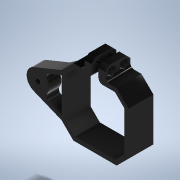
# Autodesk Inventor part: Montura motor para cadena
Saved by Autodesk Inventor 2022 (Build 260153000, 153)
## iProperties
Created: 2022-02-14
Part Number: Montura motor para cadena
Material: PET Plastic
Document SubType Name: Modeling
Designer: juanp
Density: 1.541 g/cm^3
Appearance: Polycarbonate - Clear
Author: juanp
Autodesk Inventor part; units mm, degrees
ref_plane "YZ Plane" through (0, 0, 0) normal (1, 0, 0) x (0, 1, 0)
ref_plane "XZ Plane" through (0, 0, 0) normal (0, 1, 0) x (-1, 0, 0)
ref_plane "XY Plane" through (0, 0, 0) normal (0, 0, 1) x (1, 0, 0)
sketch "Sketch1" plane through (0, 0, 0) normal (0, 0, 1) x (1, 0, 0)
  line L0 (21.15, -21.15) -> (14.4175, -21.15) construction
  line L1 (-21.15, -21.15) -> (-21.15, -14.4175) construction
  line L2 (-21.15, 21.15) -> (-14.4175, 21.15) construction
  line L3 (21.15, 21.15) -> (21.15, 14.4175) construction
  line L4 (21.15, -21.15) -> (-21.15, 21.15) construction
  line L5 (-21.15, -21.15) -> (21.15, 21.15) construction
  line L6 (-21.15, 14.4175) -> (-14.4175, 21.15) construction
  line L7 (14.4175, 21.15) -> (21.15, 14.4175) construction
  line L8 (21.15, -14.4175) -> (14.4175, -21.15) construction
  line L9 (-14.4175, -21.15) -> (-21.15, -14.4175) construction
  line L10 (-21.15, 14.4175) -> (-21.15, 21.15) construction
  line L11 (-14.4175, 21.15) -> (14.4175, 21.15) construction
  line L12 (14.4175, 21.15) -> (21.15, 21.15) construction
  line L13 (21.15, 14.4175) -> (21.15, -14.4175) construction
  line L14 (21.15, -14.4175) -> (21.15, -21.15) construction
  line L15 (14.4175, -21.15) -> (-14.4175, -21.15) construction
  line L16 (-14.4175, -21.15) -> (-21.15, -21.15) construction
  line L17 (-21.15, -14.4175) -> (-21.15, 14.4175) construction
  line L18 (-21.25, 14.4589) -> (-14.4589, 21.25)
  line L19 (-14.4589, 21.25) -> (14.4589, 21.25)
  line L20 (14.4589, 21.25) -> (21.25, 14.4589)
  line L21 (21.25, 14.4589) -> (21.25, -14.4589)
  line L22 (21.25, -14.4589) -> (14.4589, -21.25)
  line L23 (14.4589, -21.25) -> (-14.4589, -21.25)
  line L24 (-14.4589, -21.25) -> (-21.25, -14.4589)
  line L25 (-21.25, -14.4589) -> (-21.25, 14.4589)
  line L26 (-24.25, 15.7015) -> (-15.7015, 24.25)
  line L27 (-15.7015, 24.25) -> (15.7015, 24.25)
  line L28 (15.7015, 24.25) -> (24.25, 15.7015)
  line L29 (24.25, 15.7015) -> (24.25, -15.7015)
  line L30 (24.25, -15.7015) -> (15.7015, -24.25)
  line L31 (15.7015, -24.25) -> (-15.7015, -24.25)
  line L32 (-15.7015, -24.25) -> (-24.25, -15.7015)
  line L33 (-24.25, -15.7015) -> (-24.25, 15.7015)
  line L34 (-7.5, 21.25) -> (-2.5, 21.25)
  line L35 (-2.5, 21.25) -> (-2.5, 33.25)
  line L36 (-2.5, 33.25) -> (-7.5, 33.25)
  line L37 (-7.5, 33.25) -> (-7.5, 21.25)
  line L38 (2.5, 21.25) -> (7.5, 21.25)
  line L39 (7.5, 21.25) -> (7.5, 33.25)
  line L40 (7.5, 33.25) -> (2.5, 33.25)
  line L41 (2.5, 33.25) -> (2.5, 21.25)
  line L42 (-2.5, 27.25) -> (2.5, 27.25) construction
  line L43 (0, 27.25) -> (0, 21.15) construction
  point P0 (0, 0)
  point P1 (-17.7837, -17.7837)
  point P2 (-17.7837, 17.7837)
  point P3 (17.7837, 17.7837)
  point P4 (17.7837, -17.7837)
  point P5 (-7.5, 24.25)
  point P6 (7.5, 24.25)
  dimension "d0" = 42.3
  dimension "d1" = 42.3
  dimension "d2" = 50.3
  dimension "d3" = 0.1
  dimension "d4" = 3
  dimension "d5" = 5
  dimension "d6" = 5
  dimension "d7" = 9
  constraints: 88 end point, 26 parallel, 13 perpendicular, 10 midpoint, 9 point on line, 5 horizontal, 4 equal length, 1 collinear, 1 vertical, 14 other
  measures "d0" distance of L2.start L3.start
  measures "d1" distance of L1.start L2.start
  measures "d2" distance between parallel lines of L6 L8
  measures "d3" distance between parallel lines of L17 L25
  measures "d4" distance between parallel lines of L25 L33
  measures "d5" distance of L39.end L40.end
  measures "d6" distance between parallel lines of L41 L35
  measures "d7" distance between parallel lines of L40 L27
extrude "Extrusion1" add sketch "Sketch1" along normal blind 18 contours L25 L24 L23 L22 L21 L20 L19 L39 L27 L28 L29 L30 L31 L32 L33 L26 L37 L18 | L37 L27 L35 L19 | L37 L36 L35 L27 | L41 L27 L39 L19 | L41 L40 L39 L27
sketch "Sketch2" plane through (7.5, 24.25, 0) normal (1, 0, 0) x (0, 0, -1)
  line L0 (0, 0) -> (0, 9) projected
  line L1 (0, 9) -> (-18, 9) projected
  line L2 (-18, 0) -> (-18, 9) projected
  line L3 (0, 0) -> (-18, 0) projected
  line L4 (-18, 4.5) -> (-13.5, 4.5) construction
  line L5 (-4.5, 4.5) -> (0, 4.5) construction
  line L6 (0, 9) -> (0, -3) projected
  circle A0 centre (-13.5, 4.5) radius 1.65
  circle A1 centre (-4.5, 4.5) radius 1.65
  line L7 (-13.5, 4.5) -> (-9, 4.5) construction
  line L8 (-9, 4.5) -> (-4.5, 4.5) construction
  line L9 (-13.5, 1.2553) -> (-16.31, 2.8776)
  line L10 (-16.31, 2.8776) -> (-16.31, 6.1224)
  line L11 (-16.31, 6.1224) -> (-13.5, 7.7447)
  line L12 (-13.5, 7.7447) -> (-10.69, 6.1224)
  line L13 (-10.69, 6.1224) -> (-10.69, 2.8776)
  line L14 (-10.69, 2.8776) -> (-13.5, 1.2553)
  line L15 (-1.69, 2.8776) -> (-4.5, 1.2553)
  line L16 (-4.5, 1.2553) -> (-7.31, 2.8776)
  line L17 (-7.31, 2.8776) -> (-7.31, 6.1224)
  line L18 (-7.31, 6.1224) -> (-4.5, 7.7447)
  line L19 (-4.5, 7.7447) -> (-1.69, 6.1224)
  line L20 (-1.69, 6.1224) -> (-1.69, 2.8776)
  circle A2 centre (-13.5, 4.5) radius 4.5
  circle A3 centre (-4.5, 4.5) radius 4.5
  point P0 (0, -24.25)
  point P1 (-4.5, 0)
  point P2 (-13.5, 0)
  point P3 (-4.5, 9)
  point P4 (-13.5, 9)
  dimension "d10" = 3.3
  dimension "d11" = 5.62
  constraints: 32 end point, 5 coincident, 4 equal length, 3 point on line, 2 centre point, 2 horizontal, 2 vertical, 1 collinear, 1 equal radius, 1 midpoint, 1 perpendicular, 32 other
  measures "d10" diameter of A0
  measures "d11" distance between parallel lines of L10 L13
extrude "Extrusion2" cut sketch "Sketch2" against normal blind 15 contours A0 | A1
extrude "Extrusion4" cut sketch "Sketch2" against normal blind 2.35 contours L9 L10 L11 L12 L13 L14 | L15 L16 L17 L18 L19 L20
fillet "Fillet1" radius 3 4 edges at (-7.5, 24.25, 9) (2.5, 21.25, 9) (-2.5, 21.25, 9) (7.5, 24.25, 9)
chamfer "Chamfer1" distance 3 angle 45 4 edges at (-5, 33.25, 0) (5, 33.25, 0) (-5, 33.25, 18) (5, 33.25, 18)
ref_plane "Work Plane1" through (0, 0, 9) normal (0, 0, -1) x (-1, 0, 0)
sketch "Sketch3" plane through (0, 0, 9) normal (0, 0, 1) x (1, 0, 0)
  line L0 (-24.25, 15.7015) -> (-24.25, -15.7015) projected
  line L1 (-24.25, 0) -> (-41.4428, 0)
  circle A0 centre (-41.4428, 0) radius 1.65
  circle A1 centre (-41.4428, 0) radius 8.0711
  line L2 (-24.25, -15.7015) -> (-44.4822, -7.4769)
  line L3 (-24.25, 15.7015) -> (-44.4822, 7.4769)
  line L4 (-46.4428, -5) -> (-36.4428, -5)
  line L5 (-36.4428, -5) -> (-36.4428, 5)
  line L6 (-36.4428, 5) -> (-46.4428, 5)
  line L7 (-46.4428, 5) -> (-46.4428, -5)
  line L8 (-46.4428, -5) -> (-36.4428, 5) construction
  line L9 (-36.4428, -5) -> (-46.4428, 5) construction
  line L10 (-36.4428, -5) -> (-35.7357, -5.7071) construction
  line L11 (-37.5357, -7.0623) -> (-24.25, -12.4631)
  line L12 (-37.5357, 7.0623) -> (-24.25, 12.4631)
  point P0 (0, 0)
  dimension "d22" = 17.1928
  dimension "d23" = 3.3
  dimension "d27" = 10
  dimension "d28" = 10
  dimension "d35" = 1
  dimension "d36" = 3
  constraints: 24 end point, 5 point on circle, 4 parallel, 3 coincident, 3 midpoint, 2 centre point, 2 horizontal, 2 point on line, 2 tangent, 1 collinear, 1 equal length, 1 perpendicular
  measures "d22" distance of L1.start L1.end
  measures "d23" diameter of A0
  measures "d27" distance of L6.end L5.end
  measures "d28" distance of L5.end L4.end
  measures "d35" distance of L4.end L10.end
  measures "d36" distance between parallel lines of L2 L11
extrude "Extrusion5" add sketch "Sketch3" along normal blind 9 contours L0 L12 A1 L3 | A1 | A1 L11 L0 L2 | L7 L6 L5 L4
extrude "Extrusion6" add sketch "Sketch3" against normal blind 1.5 contours L7 L6 L5 L4
chamfer "Chamfer2" distance 1.5 angle 45 4 edges at (-41.4428, 5, 7.5) (-36.4428, 0, 7.5) (-41.4428, -5, 7.5) (-46.4428, 0, 7.5)
fillet "Fillet2" radius 3 2 edges at (-37.5357, -7.0623, 13.5) (-37.5357, 7.0623, 13.5)
chamfer "Chamfer4" distance 3 angle 45 2 edges at (-24.25, 14.0823, 9) (-24.25, -14.0823, 9)
body "Solid1"
